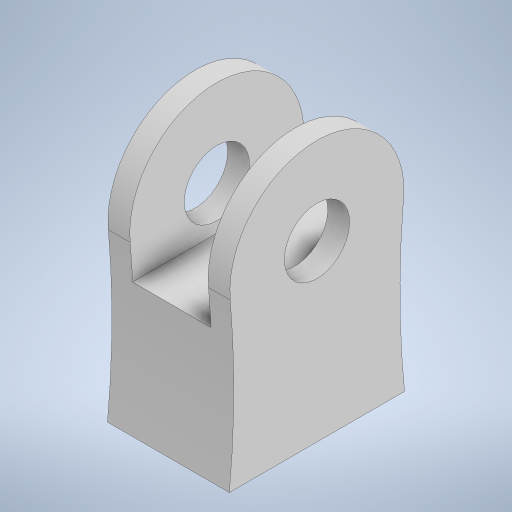
# Autodesk Inventor part: cabeza_obj1
Saved by Autodesk Inventor 2023.2 (Build 272271030, 271C)
## iProperties
Created: 2023-02-25
Part Number: cabeza_obj1
Material: Generic
Document SubType Name: Modeling
Designer: Cris Pat
Density: 1 g/cm^3
Appearance: Default
Author: Cris Pat
Autodesk Inventor part; units mm, degrees
ref_plane "YZ Plane" through (0, 0, 0) normal (1, 0, 0) x (0, 1, 0)
ref_plane "XY Plane" through (0, 0, 0) normal (0, 0, 1) x (1, 0, 0)
sketch "Sketch1" plane through (0, 0, 0) normal (1, 0, 0) x (0, 1, 0)
  circle A0 centre (0, 0) radius 7.5
  arc A1 (-3.1515, -19.7501) -> (-1.8071, 19.9182) centre (0, 0) ccw
  line L0 (-40, 20.115) -> (-40, -20.115)
  arc A2 (-40, 20.115) -> (-1.8071, 19.9182) centre (-19.8777, 219.1002) ccw
  arc A3 (-3.1515, -19.7501) -> (-40, -20.115) centre (-19.6039, -219.0723) ccw
  point P0 (-40, 0)
  dimension "d6" = 15
  dimension "d7" = 40
  dimension "d30" = 40.23
  dimension "d31" = 40
  dimension "d32" = 200
  dimension "d33" = 200
  dimension "d34" = 438.1724
  dimension "d35" = 219.0723
  constraints: 6 point on circle, 4 centre point, 3 coincident, 2 end point, 1 horizontal alignment, 1 midpoint, 1 vertical
  measures "d6" diameter of A0
  measures "d7" diameter of A1
  measures "d30" distance of L0.start L0.end
  measures "d31" distance from line of A0.centre L0
  measures "d32" radius of A2
  measures "d33" radius of A3
  measures "d34" distance of A3.centre A2.centre
  measures "d35" vertical distance of A3.centre A0.centre
extrude "Extrusion1" add sketch "Sketch1" along normal mid plane 28
sketch "Sketch3" plane through (0, 0, 0) normal (0, 0, 1) x (1, 0, 0)
  line L0 (-14, 20) -> (14, 20) construction
  line L1 (-14, -3.1515) -> (14, -3.1515) construction
  line L2 (14, -40) -> (14, -3.1515) construction
  line L3 (14, -40) -> (-14, -40) construction
  line L4 (-14, -3.1515) -> (-14, -40) construction
  line L5 (-9, 20) -> (9, 20)
  line L6 (9, 20) -> (9, -10)
  line L7 (9, -10) -> (-9, -10)
  line L8 (-9, -10) -> (-9, 20)
  point P0 (0, 0)
  point P1 (0, 20)
  point P2 (0, 20)
  dimension "d19" = 18
  dimension "d21" = 10
  constraints: 8 end point, 2 midpoint, 2 parallel, 1 coincident, 1 horizontal, 1 horizontal alignment, 1 perpendicular
  measures "d19" distance of L6.end L7.end
  measures "d21" distance from line of point (0, 0) L7
extrude "Extrusion3" cut sketch "Sketch3" along normal through all both and the other way through all
ref_plane "Work Plane1" through (0, -10, 0) normal (0, 1, 0) x (-1, 0, 0)
sketch "Sketch5" plane through (0, -10, 0) normal (0, 1, 0) x (-1, 0, 0)
  circle A0 centre (0, 0) radius 2.75
  circle A1 centre (0, 0) radius 4.3
  dimension "d37" = 5.5
  dimension "d38" = 8.6
  constraints: 2 centre point, 2 coincident
  measures "d37" diameter of A0
  measures "d38" diameter of A1
extrude "Extrusion6" cut sketch "Sketch5" against normal blind 3.2 contours A0 | A1
extrude "Extrusion7" cut sketch "Sketch5" against normal through all contours A0
body "Solid1"
